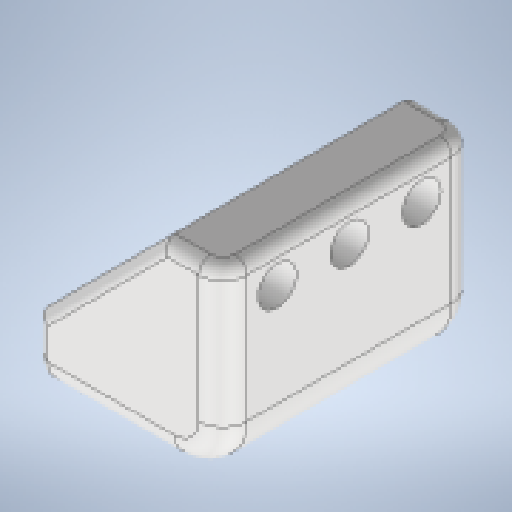
# Autodesk Inventor part: link2part3
Saved by Autodesk Inventor 2024 (Build 280153000, 153)
## iProperties
Created: 2025-02-08
Part Number: link2part3
Material: 一般
Document SubType Name: Modeling
Designer: tanoue_kota
Density: 1.0171 g/cm^3
Appearance: 既定
Mass: 3.02 g
Surface Area: 18.7893 cm^2
Volume: 2.96922 cm^3
Author: tanoue_kota
Autodesk Inventor part; units mm, degrees
ref_plane "YZ Plane" through (0, 0, 0) normal (1, 0, 0) x (0, 1, 0)
ref_plane "XZ Plane" through (0, 0, 0) normal (0, 1, 0) x (-1, 0, 0)
ref_plane "XY Plane" through (0, 0, 0) normal (0, 0, 1) x (1, 0, 0)
sketch "スケッチ1" plane through (0, 0, 0) normal (0, 0, 1) x (1, 0, 0)
  line L0 (0, 0) -> (-14, 0)
  line L1 (-14, 0) -> (-14, 14)
  line L2 (-14, 14) -> (0, 14)
  line L3 (0, 14) -> (0, 0)
  line L4 (-4, 14) -> (-14, 4)
  line L5 (-14, 4) -> (0, 4)
  line L6 (-4, 14) -> (-4, 0)
  line L7 (-4, 8) -> (-8, 4)
  dimension "d0" = 14
  dimension "d1" = 14
  dimension "d2" = 4
  dimension "d3" = 4
  dimension "d4" = 6
  constraints: 16 end point, 6 point on line, 3 parallel, 3 perpendicular, 1 horizontal
  measures "d0" distance of L1.end L2.end
  measures "d1" distance of L2.end L0.start
  measures "d2" distance from line of L3 L4.start
  measures "d3" distance from line of L0 L4.end
  measures "d4" distance from line of L2 L7.start
extrude "押し出し1" add sketch "スケッチ1" along normal blind 7 contours L0 L6 L5 L3 | L0 L1 L5 L6 | L5 L6 L2 L3 | L5 L7 L6
sketch "スケッチ2" plane through (0, 0, 7) normal (0, 0, 1) x (1, 0, 0)
  line L0 (-8, 4) -> (-14, 4) projected
  line L1 (0, 14) -> (-4, 14) projected
  line L2 (-14, 4) -> (-4, 14)
  line L3 (-4, 14) -> (0, 14)
  line L4 (0, 14) -> (0, 0)
  line L5 (0, 0) -> (-14, 0)
  line L6 (-14, 0) -> (-14, 4)
  constraints: 10 end point, 3 perpendicular, 1 collinear
extrude "押し出し2" add sketch "スケッチ2" along normal blind 1.5
mirror "ミラー1" about plane through (-7, 7, 0) normal (0, 0, -1) of "押し出し1", "押し出し2"
sketch "スケッチ3" plane through (-4, 8, 7) normal (-1, 0, 0) x (0, 0, 1)
  line L0 (-14, 6) -> (0, 6) projected
  line L1 (-7, 6) -> (-7, 0)
  line L2 (0, 0) -> (-14, 0) projected
  line L3 (-14, 6) -> (-14, 0) projected
  line L4 (-14, 3) -> (0, 3)
  line L5 (0, 6) -> (0, -4) projected
  line L6 (-15.5, -8) -> (1.5, -8) projected
  point P0 (-7, -8)
  point P1 (-7, 3)
  point P2 (-3, 3)
  point P3 (-11, 3)
  dimension "d10" = 4
  dimension "d30" = 3
  constraints: 4 end point, 4 midpoint, 2 point on line, 1 perpendicular, 1 symmetric about line
  measures "d10" distance from line of L1 point (-3, 3)
  measures "d30" distance between parallel lines of L0 L4
hole "穴1" at (-4, 11, -4) at (-4, 11, 4) direction (1, 0, 0) diameter 3.2 depth 20 tip angle 118
sketch "スケッチ4" plane through (-14, 4, 7) normal (0, 1, 0) x (1, 0, 0)
  line L0 (0, 14) -> (0, 0) projected
  line L1 (0, 7) -> (6, 7)
  line L2 (6, 14) -> (6, 0) projected
  line L3 (6, 0) -> (0, 0) projected
  line L4 (3, 0) -> (3, 14)
  line L5 (6, 14) -> (0, 14) projected
  point P0 (14, 7)
  point P1 (3, 7)
  point P2 (3, 3)
  point P3 (3, 11)
  dimension "d18" = 3
  dimension "d19" = 4
  constraints: 5 midpoint, 4 end point, 1 perpendicular, 1 point on line, 1 symmetric about line
  measures "d18" distance between parallel lines of L0 L4
  measures "d19" distance from line of L1 point (3, 3)
hole "穴2" at (-11, 4, -4) at (-11, 4, 4) direction (0, -1, 0) diameter 3.2 depth 20 tip angle 118
fillet "フィレット1" radius 4 1 edges at (0, 0, 0)
fillet "フィレット2" radius 2 6 edges at (-1.1716, 1.1716, 8.5) (0, 9, 8.5) (-9, 0, 8.5) (0, 9, -8.5) (-9, 0, -8.5) (-1.1716, 1.1716, -8.5)
fillet "フィレット3" radius 1 12 edges at (-0.5858, 14, 7.9142) (-3, 14, 8.5) (-0.5858, 14, -7.9142) (-3, 14, -8.5) (0, 14, 0) (-9, 9, 8.5) (-9, 9, -8.5) (-14, 0.5858, 7.9142) (-14, 3, 8.5) (-14, 0.5858, -7.9142) (-14, 3, -8.5) (-14, 0, 0)
